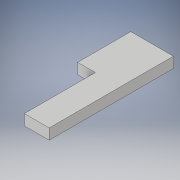
# Autodesk Inventor part: RemovableAlignmentPiece
Saved by Autodesk Inventor 2019 (Build 230136000, 136)
## iProperties
Created: 2019-06-19
Part Number: RemovableAlignmentPiece
Material: Generic
Document SubType Name: Modeling
Designer: aorfi
Density: 1 g/cm^3
Appearance: Default
Author: aorfi
Autodesk Inventor part; units mm, degrees
ref_plane "YZ Plane" through (0, 0, 0) normal (1, 0, 0) x (0, 1, 0)
ref_plane "XZ Plane" through (0, 0, 0) normal (0, 1, 0) x (-1, 0, 0)
ref_plane "XY Plane" through (0, 0, 0) normal (0, 0, 1) x (1, 0, 0)
sketch "Sketch1" plane through (0, 0, 0) normal (0, 1, 0) x (-1, 0, 0)
  line L0 (-2.5, 7.5) -> (2.5, 7.5)
  line L1 (2.5, 7.5) -> (2.5, -7.5)
  line L2 (2.5, -7.5) -> (-2.5, -7.5)
  line L3 (-2.5, -7.5) -> (-2.5, 7.5)
  line L4 (-2.5, 7.5) -> (2.5, -7.5) construction
  line L5 (2.5, 7.5) -> (-2.5, -7.5) construction
  line L6 (-2.5, -7.5) -> (-9.5, -7.5)
  line L7 (-9.5, -7.5) -> (-9.5, 27.5)
  line L8 (-9.5, 27.5) -> (-2.5, 27.5)
  line L9 (-2.5, 27.5) -> (-2.5, -7.5)
  point P0 (0, 0)
  dimension "d0" = 5
  dimension "d1" = 15
  dimension "d13" = 35
  dimension "d14" = 7
  constraints: 20 end point, 4 parallel, 2 horizontal, 2 midpoint, 2 perpendicular
  measures "d0" distance of L1.end L2.end
  measures "d1" distance of L0.end L1.end
  measures "d13" distance of L6.end L7.end
  measures "d14" distance of L7.end L8.end
extrude "Extrusion1" add sketch "Sketch1" along normal mid plane 3
sketch "Sketch3" plane through (0, -1.5, 0) normal (0, -1, 0) x (1, 0, 0)
  line L0 (1.1, 4.5) -> (-0.9, 4.5) construction
  line L1 (-0.9, 4.5) -> (-0.9, 2.5) construction
  line L2 (-0.9, 2.5) -> (1.1, 2.5) construction
  line L3 (1.1, 2.5) -> (1.1, 4.5) construction
  line L4 (1.1, 4.5) -> (-0.9, 2.5) construction
  line L5 (-0.9, 4.5) -> (1.1, 2.5) construction
  line L6 (1.1, -2.5) -> (-0.9, -2.5) construction
  line L7 (-0.9, -2.5) -> (-0.9, -4.5) construction
  line L8 (-0.9, -4.5) -> (1.1, -4.5) construction
  line L9 (1.1, -4.5) -> (1.1, -2.5) construction
  line L10 (1.1, -2.5) -> (-0.9, -4.5) construction
  line L11 (-0.9, -2.5) -> (1.1, -4.5) construction
  line L12 (0.1, 3.5) -> (0.1, -3.5) construction
  line L13 (-2.5, -7.5) -> (9.5, -7.5) construction
  line L14 (1.05, 2.55) -> (-0.85, 2.55)
  line L15 (-0.85, 2.55) -> (-0.85, 4.45)
  line L16 (-0.85, 4.45) -> (1.05, 4.45)
  line L17 (1.05, 4.45) -> (1.05, 2.55)
  line L18 (-0.85, -2.55) -> (1.05, -2.55)
  line L19 (1.05, -2.55) -> (1.05, -4.45)
  line L20 (1.05, -4.45) -> (-0.85, -4.45)
  line L21 (-0.85, -4.45) -> (-0.85, -2.55)
  line L22 (-2.5, 7.5) -> (-2.5, -7.5) projected
  point P0 (0, 0)
  point P1 (0.1, 0)
  dimension "d7" = 2
  dimension "d8" = 7
  dimension "d11" = 0.05
  dimension "d12" = 0.05
  dimension "d18" = 2.6
  constraints: 42 end point, 8 parallel, 5 midpoint, 4 perpendicular, 3 equal length, 2 horizontal, 1 horizontal alignment, 1 point on line, 1 vertical, 6 other
  measures "d7" distance of L2.end L0.start
  measures "d8" distance of L12.start L12.end
  measures "d11" distance between parallel lines of L2 L14
  measures "d12" distance between parallel lines of L6 L18
  measures "d18" distance from line of L22 L12.end
extrude "Extrusion3" add sketch "Sketch3" along normal blind 2
body "Solid1"
